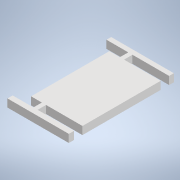
# Autodesk Inventor part: bottom
Saved by Autodesk Inventor 2020.2 (Build 242310000, 310)
## iProperties
Created: 2020-03-18
Part Number: bottom
Material: Generic
Document SubType Name: Modeling
Designer: deli
Density: 1 g/cm^3
Appearance: Default
Author: deli
Autodesk Inventor part; units mm, degrees
ref_plane "YZ Plane" through (0, 0, 0) normal (1, 0, 0) x (0, 1, 0)
ref_plane "XZ Plane" through (0, 0, 0) normal (0, 1, 0) x (-1, 0, 0)
ref_plane "XY Plane" through (0, 0, 0) normal (0, 0, 1) x (1, 0, 0)
sketch "Sketch1" plane through (0, 0, 0) normal (0, 1, 0) x (-1, 0, 0)
  line L0 (-19.5047, -110.1246) -> (-72.2097, -110.1246)
  line L1 (-72.2097, -110.1246) -> (-72.2097, -89.8046)
  line L2 (-46.8097, -89.8046) -> (-72.2097, -89.8046)
  line L3 (-82.3697, -110.1246) -> (-171.0229, -110.1246)
  line L4 (-82.3697, -89.8046) -> (-171.0229, -89.8046)
  line L5 (-82.3697, -110.1246) -> (-82.3697, -89.8046)
  line L6 (-171.0229, -121.5546) -> (-19.5047, -121.5546)
  line L7 (-19.5047, -121.5546) -> (-19.5047, -110.1246)
  line L8 (-46.8097, 99.4254) -> (-46.8097, -89.8046)
  line L9 (-72.8447, 99.4254) -> (-72.8447, 119.7454)
  line L10 (-72.8447, 119.7454) -> (-22.6797, 119.7454)
  line L11 (-83.0047, 99.4254) -> (-83.0047, 119.7454)
  line L12 (-83.0047, 119.7454) -> (-171.0229, 119.7454)
  line L13 (-171.0229, 132.4454) -> (-22.6797, 132.4454)
  line L14 (-22.6797, 132.4454) -> (-22.6797, 119.7454)
  line L15 (-171.0229, 99.4254) -> (-83.0047, 99.4254)
  line L16 (-72.8447, 99.4254) -> (-46.8097, 99.4254)
  line L17 (-22.6797, 119.7454) -> (-72.8447, 119.7454)
  line L18 (-83.0047, 119.7454) -> (-171.0229, 119.7454)
  line L19 (-171.0229, 132.4454) -> (-171.0229, 119.7454)
  line L20 (-171.0229, 99.4254) -> (-171.0229, -89.8046)
  line L21 (-171.0229, -110.1246) -> (-171.0229, -121.5546)
  point P0 (0, 0)
  dimension "d3" = 20.32
  dimension "d4" = 20.32
  dimension "d6" = 254
  dimension "d7" = 0
  dimension "d10" = 20.32
  dimension "d11" = 20.32
  dimension "d12" = 0
  dimension "d13" = 10.16
  dimension "d14" = 26.035
  dimension "d16" = 25.4
  dimension "d17" = 10.16
  constraints: 48 end point, 2 horizontal, 2 parallel
  measures "d3" distance of L9.start L9.end
  measures "d4" distance of L11.end L11.start
  measures "d6" distance between parallel lines of L13 L6
  measures "d7" distance between parallel lines of L15 L16
  measures "d10" distance between parallel lines of L3 L4
  measures "d11" distance between parallel lines of L0 L2
  measures "d12" distance between parallel lines of L4 L2
  measures "d13" distance between parallel lines of L11 L9
  measures "d14" distance between parallel lines of L9 L8
  measures "d16" distance between parallel lines of L1 L8
  measures "d17" distance between parallel lines of L5 L1
extrude "Extrusion1" add sketch "Sketch1" along normal blind 19.05
equation "\"d4\" = d3"
equation "\"d10\" = d4"
equation "\"d11\" = d3"
equation "\"d17\" = d13"
body "Solid1"
